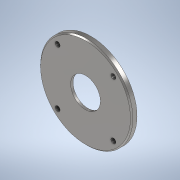
# Autodesk Inventor part: МПСТ Крышка подшипника с отверстием 110
Saved by Autodesk Inventor 2022.1 (Build 261234020, 234B)
## iProperties
Created: 2021-12-16
Part Number: МПСТ Крышка подшипника с отверстием 110
Material: Сталь, углеродистая
Document SubType Name: Modeling
Designer: Алексанян Г.
Density: 7.85 g/cm^3
Appearance: С умеренной полировкой
Author: Алексанян Г.
Autodesk Inventor part; units mm, degrees
ref_plane "YZ Plane" through (0, 0, 0) normal (1, 0, 0) x (0, 1, 0)
ref_plane "XZ Plane" through (0, 0, 0) normal (0, 1, 0) x (-1, 0, 0)
ref_plane "XY Plane" through (0, 0, 0) normal (0, 0, 1) x (1, 0, 0)
sketch "Эскиз1" plane through (0, 0, 0) normal (0, 1, 0) x (-1, 0, 0)
  line L0 (0, 0) -> (77.5, 0)
  line L1 (77.5, 0) -> (77.5, -9)
  line L2 (77.5, -9) -> (55, -9)
  line L3 (55, -9) -> (55, -15)
  line L4 (0, -4) -> (0, 0)
  line L5 (55, -15) -> (45, -15)
  line L6 (45, -15) -> (45, -4)
  line L7 (45, -4) -> (0, -4)
  dimension "d0" = 155
  dimension "d1" = 110
  dimension "d3" = 9
  dimension "d5" = 15
  dimension "d6" = 90
  dimension "d7" = 4
  constraints: 17 end point, 5 perpendicular, 2 horizontal, 1 vertical
  measures "d0" diameter of L1 L4
  measures "d1" diameter of L3 L4
  measures "d3" distance between parallel lines of L0 L2
  measures "d5" distance between parallel lines of L0 L5
  measures "d6" diameter of L6 L4
  measures "d7" distance between parallel lines of L0 L7
revolve "Вращение1" add sketch "Эскиз1" angle 360 about axis through (0, 0, -4) along (0, 0, 1)
sketch "Эскиз3" plane through (0, 0, 0) normal (0, 0, 1) x (1, 0, 0)
  circle A0 centre (0, 0) radius 66.25 construction
  line L0 (0, 0) -> (-70.023, -70.023) construction
  line L1 (0, 0) -> (99.0274, 0) construction
  point P0 (0, 0)
  point P1 (-46.8458, -46.8458)
  point P2 (46.8458, -46.8458)
  point P3 (46.8458, 46.8458)
  point P4 (-46.8458, 46.8458)
  dimension "d15" = 132.5
  dimension "d16" = 135
  dimension "d19" = 360
  constraints: 4 end point, 1 coincident, 1 equal length, 1 horizontal, 1 point on line, 8 other
  measures "d16" angle of L0 L1
hole "Отверстие1" at (-46.8458, -46.8458, 0) at (46.8458, -46.8458, 0) at (46.8458, 46.8458, 0) at (-46.8458, 46.8458, 0) direction (0, 0, -1) diameter 8.376 end through all thread size "M10x1.5" class "6H" standard "ISO Metric profile"
chamfer "Фаска1" distance 2 angle 45 2 edges at (55, 0, -15) (77.5, 0, 0)
sketch "Эскиз4" plane through (0, 0, 0) normal (0, 0, 1) x (1, 0, 0)
  circle A0 centre (0, 0) radius 77.5 projected
  point P0 (0, 0)
  constraints: 1 coincident
hole "Отверстие2" at (0, 0, 0) direction (0, 0, -1) diameter 50 end through all
